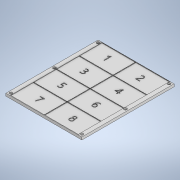
# Autodesk Inventor part: 8pos_slas_table
Saved by Autodesk Inventor 2020 (Build 240168000, 168)
## iProperties
Created: 2023-04-21
Part Number: 8pos_slas_table
Material: Generic
Document SubType Name: Modeling
Designer: Beaucage
Density: 1 g/cm^3
Appearance: Default
Author: Beaucage
Autodesk Inventor part; units mm, degrees
ref_plane "YZ Plane" through (0, 0, 0) normal (1, 0, 0) x (0, 1, 0)
ref_plane "XZ Plane" through (0, 0, 0) normal (0, 1, 0) x (-1, 0, 0)
ref_plane "XY Plane" through (0, 0, 0) normal (0, 0, 1) x (1, 0, 0)
sketch "Sketch1" plane through (0, 0, 0) normal (0, 1, 0) x (-1, 0, 0)
  line L0 (0, 0) -> (290, 0)
  line L1 (290, 0) -> (290, -351.8916)
  line L2 (290, -351.8916) -> (0, -351.8916)
  line L3 (0, -351.8916) -> (0, 0)
  dimension "d0" = 290
  dimension "d1" = 351.8916
  constraints: 8 end point, 2 parallel, 1 horizontal, 1 perpendicular
  measures "d0" distance of L1.end L2.end
  measures "d1" distance of L0.end L1.end
extrude "Extrusion1" add sketch "Sketch1" along normal blind 10
sketch "Sketch2" plane through (0, 10, 0) normal (0, 1, 0) x (1, 0, 0)
  line L0 (-290, 0) -> (0, 0) projected
  line L1 (0, 0) -> (-2, 0)
  line L2 (-2, 0) -> (-2, 2)
  line L3 (-2, 2) -> (0, 2)
  line L4 (0, 2) -> (0, 0)
  line L5 (0, 0) -> (0, 351.8916) projected
  line L6 (-2, 2) -> (0, 2)
  line L7 (0, 2) -> (0, 351.8916)
  line L8 (0, 351.8916) -> (-2, 351.8916)
  line L9 (-2, 351.8916) -> (-2, 2)
  line L10 (-290, 351.8916) -> (-290, 0) projected
  line L11 (0, 351.8916) -> (-290, 351.8916)
  line L12 (-290, 351.8916) -> (-290, 349.8916)
  line L13 (-290, 349.8916) -> (0, 349.8916)
  line L14 (0, 349.8916) -> (0, 351.8916)
  line L15 (0, 351.8916) -> (-290, 351.8916) projected
  line L16 (-290, 351.8916) -> (-288, 351.8916)
  line L17 (-288, 351.8916) -> (-288, 0)
  line L18 (-288, 0) -> (-290, 0)
  line L19 (-290, 0) -> (-290, 351.8916)
  line L20 (-290, 0) -> (0, 0)
  line L21 (0, 0) -> (0, 2)
  line L22 (0, 2) -> (-290, 2)
  line L23 (-290, 2) -> (-290, 0)
  line L24 (-2, 2) -> (-129.762, 2)
  line L25 (-2, 87.471) -> (-2, 2)
  line L26 (-131.762, 2) -> (-129.762, 2)
  line L27 (-288, 87.471) -> (-288, 89.471)
  line L28 (-2, 89.471) -> (-2, 87.471)
  line L29 (-262.0386, 2) -> (-134.2766, 2)
  line L30 (0, 2) -> (-15.7353, 2)
  line L31 (-15.7353, 2) -> (-144.5133, 2)
  line L32 (-144.5133, 2) -> (-144.5133, 88.487)
  line L33 (-144.5133, 88.487) -> (-15.7353, 88.487)
  line L34 (-15.7353, 88.487) -> (-15.7353, 2)
  line L35 (-144.5133, 88.487) -> (-146.5133, 88.487)
  line L36 (-146.5133, 88.487) -> (-146.5133, 2)
  line L37 (-146.5133, 2) -> (-144.5133, 2)
  line L38 (-144.5133, 2) -> (-144.5133, 88.487)
  point P0 (-288, 2)
  point P1 (-2, 349.8916)
  point P2 (-288, 349.8916)
  point P3 (-144.5133, 2)
  point P4 (-15.7353, 2)
  dimension "d4" = 2
  dimension "d5" = 2
  dimension "d6" = 2
  dimension "d7" = 2
  dimension "d8" = 2
  dimension "d13" = 2
  dimension "d14" = 2
  dimension "d17" = 127.762
  dimension "d19" = 15.7353
  dimension "d20" = 128.778
  dimension "d21" = 86.487
  dimension "d22" = 2
  constraints: 70 end point, 15 parallel, 8 horizontal, 7 perpendicular, 6 point on line
  measures "d4" distance of L2.end L3.end
  measures "d5" distance of L1.end L2.end
  measures "d6" distance of L12.end L11.end
  measures "d7" distance of L17.end L18.end
  measures "d8" distance of L6.end L20.end
  measures "d13" distance of L26.end L26.start
  measures "d14" distance of L27.start L27.end
  measures "d17" distance of L29.end L29.start
  measures "d19" distance of L6.end L30.end
  measures "d20" distance of L32.end L33.end
  measures "d21" distance of L31.end L32.end
  measures "d22" distance of L37.end L36.end
extrude "Extrusion4" cut sketch "Sketch2" against normal blind 2 contours L22 L32 L33 L34
pattern_linear "Rectangular Pattern1" count 2 spacing 129.762 along (-1, 0, 0) count 4 spacing 87.471 along (0, 0, -1) of "Extrusion4"
sketch "Sketch3" plane through (0, 10, 0) normal (0, 1, 0) x (1, 0, 0)
  line L0 (-290, 351.8916) -> (-290, 0) projected
  line L1 (-290, 0) -> (-280.475, 0)
  line L2 (-290, 0) -> (0, 0) projected
  line L3 (-280.475, 0) -> (-280.475, 9.525)
  line L4 (-290, 351.8916) -> (-280.475, 351.8916)
  line L5 (-280.475, 351.8916) -> (-280.475, 342.3666)
  line L6 (0, 0) -> (0, 351.8916) projected
  line L7 (0, 351.8916) -> (-9.525, 351.8916)
  line L8 (0, 351.8916) -> (-290, 351.8916) projected
  line L9 (-9.525, 351.8916) -> (-9.525, 342.3666)
  line L10 (0, 0) -> (-9.525, 0)
  line L11 (-9.525, 0) -> (-9.525, 9.525)
  line L12 (-290, 351.8916) -> (-290, 0) projected
  line L13 (-290, 175.9458) -> (-280.475, 175.9458)
  line L14 (0, 175.9458) -> (-9.525, 175.9458)
  dimension "d31" = 9.525
  dimension "d32" = 9.525
  dimension "d33" = 9.525
  dimension "d34" = 9.525
  dimension "d35" = 9.525
  dimension "d36" = 9.525
  constraints: 20 end point, 3 horizontal, 3 perpendicular, 3 point on line, 2 midpoint, 1 vertical
  measures "d31" distance of L0.end L1.end
  measures "d32" distance of L1.end L3.end
  measures "d33" distance of L0.start L4.end
  measures "d34" distance of L4.end L5.end
  measures "d35" distance of L6.end L7.end
  measures "d36" distance of L10.end L11.end
hole "Hole1" at (-280.475, 10, -342.3666) at (-9.525, 10, -342.3666) at (-9.525, 10, -9.525) at (-280.475, 10, -9.525) at (-280.475, 10, -175.9458) at (-9.525, 10, -175.9458) direction (0, -1, 0) diameter 6.7564 depth 9.9 counterbore diameter 11.1252 counterbore depth 6.35 clearance for "Socket Head Cap Screw" size "1/4" standard "Ansi Unified Screw Threads"
sketch "Sketch4" plane through (0, 8, 0) normal (0, 1, 0) x (1, 0, 0)
  line L0 (-94.0241, 322.1663) -> (-46.4018, 322.1663) construction
  line L1 (-46.4018, 322.1663) -> (-46.4018, 267.8366) construction
  line L2 (-46.4018, 267.8366) -> (-94.0241, 267.8366) construction
  line L3 (-94.0241, 267.8366) -> (-94.0241, 322.1663) construction
  line L4 (-224.5716, 324.4245) -> (-176.9493, 324.4245) construction
  line L5 (-176.9493, 324.4245) -> (-176.9493, 270.0949) construction
  line L6 (-176.9493, 270.0949) -> (-224.5716, 270.0949) construction
  line L7 (-224.5716, 270.0949) -> (-224.5716, 324.4245) construction
  line L8 (-224.5716, 324.4245) -> (-176.9493, 324.4245) construction
  line L9 (-176.9493, 324.4245) -> (-176.9493, 270.0949) construction
  line L10 (-176.9493, 270.0949) -> (-224.5716, 270.0949) construction
  line L11 (-224.5716, 270.0949) -> (-224.5716, 324.4245) construction
  line L12 (-223.2301, 237.2288) -> (-175.6078, 237.2288) construction
  line L13 (-175.6078, 237.2288) -> (-175.6078, 182.8992) construction
  line L14 (-175.6078, 182.8992) -> (-223.2301, 182.8992) construction
  line L15 (-223.2301, 182.8992) -> (-223.2301, 237.2288) construction
  line L16 (-92.8613, 183.1452) -> (-92.8613, 237.4748) construction
  line L17 (-92.8613, 237.4748) -> (-45.239, 237.4748) construction
  line L18 (-45.239, 237.4748) -> (-45.239, 183.1452) construction
  line L19 (-45.239, 183.1452) -> (-92.8613, 183.1452) construction
  line L20 (-91.7658, 148.6916) -> (-44.1436, 148.6916) construction
  line L21 (-44.1436, 148.6916) -> (-44.1436, 94.362) construction
  line L22 (-44.1436, 94.362) -> (-91.7658, 94.362) construction
  line L23 (-91.7658, 94.362) -> (-91.7658, 148.6916) construction
  line L24 (-220.3011, 93.2666) -> (-220.3011, 147.5962) construction
  line L25 (-220.3011, 147.5962) -> (-172.6789, 147.5962) construction
  line L26 (-172.6789, 147.5962) -> (-172.6789, 93.2666) construction
  line L27 (-172.6789, 93.2666) -> (-220.3011, 93.2666) construction
  line L28 (-216.9474, 3.3879) -> (-216.9474, 57.7176) construction
  line L29 (-216.9474, 57.7176) -> (-169.3252, 57.7176) construction
  line L30 (-169.3252, 57.7176) -> (-169.3252, 3.3879) construction
  line L31 (-169.3252, 3.3879) -> (-216.9474, 3.3879) construction
  line L32 (-89.2616, 4.3047) -> (-89.2616, 58.6343) construction
  line L33 (-89.2616, 58.6343) -> (-41.6393, 58.6343) construction
  line L34 (-41.6393, 58.6343) -> (-41.6393, 4.3047) construction
  line L35 (-41.6393, 4.3047) -> (-89.2616, 4.3047) construction
  spline S0 degree 2 poles (-87.6593, 39.9024) (-87.6593, 40.9156) (-87.0232, 42.9419) (-85.845, 44.7091) (-84.0779, 46.17) (-82.9705, 46.5941) knots 0 0 0 1 2 3 4 4 4
  spline S1 degree 2 poles (-82.9705, 46.5941) (-84.6198, 47.513) (-86.5755, 50.4111) (-86.5755, 52.1547) knots 0 0 0 1 2 2 2
  spline S2 degree 2 poles (-86.5755, 52.1547) (-86.5755, 53.5685) (-85.4916, 55.9247) (-83.5831, 57.6683) (-80.9441, 58.6343) (-79.4361, 58.6343) knots 0 0 0 1 2 3 4 4 4
  spline S3 degree 2 poles (-79.4361, 58.6343) (-77.881, 58.6343) (-75.2656, 57.6447) (-73.3571, 55.9247) (-72.2968, 53.5449) (-72.2968, 52.1547) knots 0 0 0 1 2 3 4 4 4
  spline S4 degree 2 poles (-72.2968, 52.1547) (-72.2968, 50.4111) (-74.2289, 47.513) (-75.8547, 46.5941) knots 0 0 0 1 2 2 2
  spline S5 degree 2 poles (-75.8547, 46.5941) (-74.7473, 46.17) (-73.0037, 44.7091) (-71.8256, 42.9419) (-71.1894, 40.9156) (-71.1894, 39.9024) knots 0 0 0 1 2 3 4 4 4
  spline S6 degree 2 poles (-71.1894, 39.9024) (-71.1894, 38.2295) (-72.3911, 35.4727) (-74.5823, 33.4935) (-77.5983, 32.4097) (-79.4361, 32.4097) knots 0 0 0 1 2 3 4 4 4
  spline S7 degree 2 poles (-79.4361, 32.4097) (-81.2269, 32.4097) (-84.2428, 33.4935) (-86.4341, 35.4727) (-87.6593, 38.2295) (-87.6593, 39.9024) knots 0 0 0 1 2 3 4 4 4
  spline S8 degree 2 poles (-84.502, 40.138) (-84.502, 38.9599) (-83.7951, 37.0514) (-82.4521, 35.7084) (-80.5671, 34.9779) (-79.4126, 34.9779) knots 0 0 0 1 2 3 4 4 4
  spline S9 degree 2 poles (-79.4126, 34.9779) (-78.3052, 34.9779) (-76.4202, 35.7084) (-75.0536, 37.0514) (-74.2996, 38.9835) (-74.2996, 40.138) knots 0 0 0 1 2 3 4 4 4
  spline S10 degree 2 poles (-74.2996, 40.138) (-74.2996, 41.1983) (-75.0065, 43.0598) (-76.3731, 44.497) (-78.2345, 45.2982) (-79.4126, 45.2982) knots 0 0 0 1 2 3 4 4 4
  spline S11 degree 2 poles (-79.4126, 45.2982) (-80.52, 45.2982) (-82.3578, 44.5442) (-83.7245, 43.1776) (-84.502, 41.269) (-84.502, 40.138) knots 0 0 0 1 2 3 4 4 4
  spline S12 degree 2 poles (-83.6066, 51.9191) (-83.6066, 51.0238) (-82.9469, 49.4922) (-81.7924, 48.3377) (-80.2844, 47.6779) (-79.4126, 47.6779) knots 0 0 0 1 2 3 4 4 4
  spline S13 degree 2 poles (-79.4126, 47.6779) (-78.5408, 47.6779) (-77.0092, 48.3377) (-75.8783, 49.4922) (-75.195, 51.0473) (-75.195, 51.9191) knots 0 0 0 1 2 3 4 4 4
  spline S14 degree 2 poles (-75.195, 51.9191) (-75.195, 52.838) (-75.8547, 54.4167) (-76.9857, 55.5477) (-78.5172, 56.2074) (-79.4126, 56.2074) knots 0 0 0 1 2 3 4 4 4
  spline S15 degree 2 poles (-79.4126, 56.2074) (-80.3551, 56.2074) (-81.8866, 55.5241) (-83.0176, 54.3696) (-83.6066, 52.8145) (-83.6066, 51.9191) knots 0 0 0 1 2 3 4 4 4
  spline S16 degree 2 poles (-199.0638, 56.0447) (-199.6293, 55.0315) (-201.2786, 52.0155) (-203.1165, 48.2691) (-205.0486, 43.9337) (-206.6979, 39.3391) (-207.9703, 34.6031) (-208.253, 32.3176) knots 0 0 0 1 2 3 4 5 6 6 6
  line L36 (-208.253, 32.3176) -> (-211.3632, 32.3176)
  spline S17 degree 2 poles (-211.3632, 32.3176) (-211.0569, 34.5795) (-209.7139, 39.3155) (-208.0409, 43.863) (-206.156, 48.0806) (-204.3888, 51.6385) (-202.9044, 54.3482) (-202.4803, 55.1022) knots 0 0 0 1 2 3 4 5 6 6 6
  line L37 (-202.4803, 55.1022) -> (-215.2038, 55.1022)
  line L38 (-215.2038, 55.1022) -> (-215.2038, 57.7176)
  line L39 (-215.2038, 57.7176) -> (-199.0638, 57.7176)
  line L40 (-199.0638, 57.7176) -> (-199.0638, 56.0447)
  spline S18 degree 2 poles (-203.1243, 129.9482) (-203.1243, 128.0867) (-204.3967, 125.0943) (-206.7529, 122.9266) (-210.0987, 121.7485) (-212.1251, 121.7485) knots 0 0 0 1 2 3 4 4 4
  spline S19 degree 2 poles (-212.1251, 121.7485) (-215.6829, 121.7485) (-217.403, 122.8088) knots 0 0 0 1 1 1
  line L41 (-217.403, 122.8088) -> (-217.403, 125.8955)
  spline S20 degree 2 poles (-217.403, 125.8955) (-214.8111, 124.2225) (-212.1015, 124.2225) knots 0 0 0 1 1 1
  spline S21 degree 2 poles (-212.1015, 124.2225) (-210.7113, 124.2225) (-208.4965, 125.0472) (-206.9414, 126.5081) (-206.1167, 128.558) (-206.1167, 129.7832) knots 0 0 0 1 2 3 4 4 4
  spline S22 degree 2 poles (-206.1167, 129.7832) (-206.1167, 132.2572) (-209.439, 135.0847) (-212.6199, 135.0847) knots 0 0 0 1 2 2 2
  spline S23 degree 2 poles (-212.6199, 135.0847) (-213.1147, 135.0847) (-214.2692, 135.0376) (-215.4002, 134.9905) (-216.4841, 134.9198) (-216.9082, 134.8726) knots 0 0 0 1 2 3 4 4 4
  line L42 (-216.9082, 134.8726) -> (-216.0599, 147.5962)
  line L43 (-216.0599, 147.5962) -> (-204.3024, 147.5962)
  line L44 (-204.3024, 147.5962) -> (-204.3024, 144.9808)
  line L45 (-204.3024, 144.9808) -> (-213.5388, 144.9808)
  line L46 (-213.5388, 144.9808) -> (-214.0572, 137.5116)
  spline S24 degree 2 poles (-214.0572, 137.5116) (-213.4681, 137.5587) (-212.1957, 137.6058) (-211.7009, 137.6058) knots 0 0 0 1 2 2 2
  spline S25 degree 2 poles (-211.7009, 137.6058) (-209.6982, 137.6058) (-206.4937, 136.5456) (-204.2789, 134.5899) (-203.1243, 131.7389) (-203.1243, 129.9482) knots 0 0 0 1 2 3 4 4 4
  spline S26 degree 2 poles (-73.6465, 130.9258) (-73.6465, 129.0644) (-74.8718, 125.9542) (-76.9924, 123.6922) (-79.9376, 122.4198) (-81.6577, 122.4198) knots 0 0 0 1 2 3 4 4 4
  spline S27 degree 2 poles (-81.6577, 122.4198) (-83.5662, 122.4198) (-86.5821, 124.0221) (-88.7027, 127.0145) (-89.8102, 131.3263) (-89.8102, 134.036) knots 0 0 0 1 2 3 4 4 4
  spline S28 degree 2 poles (-89.8102, 134.036) (-89.8102, 137.3583) (-88.3257, 142.754) (-85.6161, 146.6182) (-81.799, 148.6916) (-79.4428, 148.6916) knots 0 0 0 1 2 3 4 4 4
  spline S29 degree 2 poles (-79.4428, 148.6916) (-76.8039, 148.6916) (-75.2252, 147.9848) knots 0 0 0 1 1 1
  line L47 (-75.2252, 147.9848) -> (-75.2252, 145.228)
  spline S30 degree 2 poles (-75.2252, 145.228) (-77.1808, 146.2412) (-79.3721, 146.2412) knots 0 0 0 1 1 1
  spline S31 degree 2 poles (-79.3721, 146.2412) (-81.0686, 146.2412) (-83.8018, 144.7096) (-85.7339, 141.9293) (-86.7942, 137.9944) (-86.7942, 135.5911) knots 0 0 0 1 2 3 4 4 4
  line L48 (-86.7942, 135.5911) -> (-86.7235, 135.5911)
  spline S32 degree 2 poles (-86.7235, 135.5911) (-84.9564, 138.772) (-80.9272, 138.772) knots 0 0 0 1 1 1
  spline S33 degree 2 poles (-80.9272, 138.772) (-79.2543, 138.772) (-76.5918, 137.6174) (-74.6833, 135.544) (-73.6465, 132.6929) (-73.6465, 130.9258) knots 0 0 0 1 2 3 4 4 4
  spline S34 degree 2 poles (-76.6389, 130.5488) (-76.6389, 131.8918) (-77.2987, 134.0124) (-78.571, 135.4968) (-80.4089, 136.298) (-81.587, 136.298) knots 0 0 0 1 2 3 4 4 4
  spline S35 degree 2 poles (-81.587, 136.298) (-82.6473, 136.298) (-84.5087, 135.4733) (-85.8517, 134.0831) (-86.6057, 132.2217) (-86.6057, 131.185) knots 0 0 0 1 2 3 4 4 4
  spline S36 degree 2 poles (-86.6057, 131.185) (-86.6057, 129.8655) (-85.8753, 127.58) (-84.5087, 125.8835) (-82.6473, 124.8939) (-81.5163, 124.8939) knots 0 0 0 1 2 3 4 4 4
  spline S37 degree 2 poles (-81.5163, 124.8939) (-80.4324, 124.8939) (-78.6181, 125.7421) (-77.3458, 127.2265) (-76.6389, 129.3) (-76.6389, 130.5488) knots 0 0 0 1 2 3 4 4 4
  line L49 (-77.805, 237.4748) -> (-77.805, 220.6986)
  line L50 (-77.805, 220.6986) -> (-74.5299, 220.6986)
  line L51 (-74.5299, 220.6986) -> (-74.5299, 218.0361)
  line L52 (-74.5299, 218.0361) -> (-77.805, 218.0361)
  line L53 (-77.805, 218.0361) -> (-77.805, 212.0748)
  line L54 (-77.805, 212.0748) -> (-80.6796, 212.0748)
  line L55 (-80.6796, 212.0748) -> (-80.6796, 218.0361)
  line L56 (-80.6796, 218.0361) -> (-92.6021, 218.0361)
  line L57 (-92.6021, 218.0361) -> (-92.6021, 220.5572)
  spline S38 degree 2 poles (-92.6021, 220.5572) (-90.9527, 222.4422) (-87.5362, 226.7069) (-84.4496, 231.1131) (-81.8106, 235.4721) (-80.8917, 237.4748) knots 0 0 0 1 2 3 4 4 4
  line L58 (-80.8917, 237.4748) -> (-77.805, 237.4748)
  line L59 (-89.3269, 220.6986) -> (-80.6796, 220.6986)
  line L60 (-80.6796, 220.6986) -> (-80.6796, 233.1394)
  spline S39 degree 2 poles (-80.6796, 233.1394) (-81.9991, 230.8303) (-84.3789, 227.1782) (-86.523, 224.1858) (-88.4787, 221.7824) (-89.3269, 220.6986) knots 0 0 0 1 2 3 4 4 4
  spline S40 degree 2 poles (-206.336, 218.5911) (-206.336, 216.8711) (-207.632, 214.0672) (-209.9882, 212.0644) (-213.2869, 210.957) (-215.2661, 210.957) knots 0 0 0 1 2 3 4 4 4
  spline S41 degree 2 poles (-215.2661, 210.957) (-218.9182, 210.957) (-221.0624, 212.3472) knots 0 0 0 1 1 1
  line L61 (-221.0624, 212.3472) -> (-221.0624, 215.4574)
  spline S42 degree 2 poles (-221.0624, 215.4574) (-218.4705, 213.431) (-215.1718, 213.431) knots 0 0 0 1 1 1
  spline S43 degree 2 poles (-215.1718, 213.431) (-213.8288, 213.431) (-211.6846, 214.1143) (-210.1531, 215.3867) (-209.3284, 217.201) (-209.3284, 218.332) knots 0 0 0 1 2 3 4 4 4
  spline S44 degree 2 poles (-209.3284, 218.332) (-209.3284, 223.3036) (-216.3971, 223.3036) knots 0 0 0 1 1 1
  line L62 (-216.3971, 223.3036) -> (-218.5177, 223.3036)
  line L63 (-218.5177, 223.3036) -> (-218.5177, 225.7776)
  line L64 (-218.5177, 225.7776) -> (-216.5149, 225.7776)
  spline S45 degree 2 poles (-216.5149, 225.7776) (-210.2474, 225.7776) (-210.2474, 230.4429) knots 0 0 0 1 1 1
  spline S46 degree 2 poles (-210.2474, 230.4429) (-210.2474, 234.7783) (-215.0305, 234.7783) knots 0 0 0 1 1 1
  spline S47 degree 2 poles (-215.0305, 234.7783) (-217.7166, 234.7783) (-220.0728, 232.9641) knots 0 0 0 1 1 1
  line L65 (-220.0728, 232.9641) -> (-220.0728, 235.7915)
  spline S48 degree 2 poles (-220.0728, 235.7915) (-217.6459, 237.2288) (-214.3, 237.2288) knots 0 0 0 1 1 1
  spline S49 degree 2 poles (-214.3, 237.2288) (-212.6978, 237.2288) (-210.1295, 236.357) (-208.2681, 234.7548) (-207.255, 232.5164) (-207.255, 231.1733) knots 0 0 0 1 2 3 4 4 4
  spline S50 degree 2 poles (-207.255, 231.1733) (-207.255, 226.1546) (-212.3444, 224.7173) knots 0 0 0 1 1 1
  line L66 (-212.3444, 224.7173) -> (-212.3444, 224.6466)
  spline S51 degree 2 poles (-212.3444, 224.6466) (-211.0485, 224.5052) (-208.8336, 223.5392) (-207.255, 221.9841) (-206.336, 219.8635) (-206.336, 218.5911) knots 0 0 0 1 2 3 4 4 4
  line L67 (-211.7538, 298.459) -> (-214.6519, 298.459)
  line L68 (-214.6519, 298.459) -> (-214.6519, 320.4189)
  spline S52 degree 2 poles (-214.6519, 320.4189) (-214.9818, 320.0655) (-216.2777, 319.2173) (-217.9035, 318.3455) (-219.6706, 317.615) (-220.5424, 317.403) knots 0 0 0 1 2 3 4 4 4
  line L69 (-220.5424, 317.403) -> (-220.5424, 320.3482)
  spline S53 degree 2 poles (-220.5424, 320.3482) (-219.5764, 320.6074) (-217.4322, 321.5028) (-215.3588, 322.6338) (-213.5209, 323.859) (-212.8376, 324.4245) knots 0 0 0 1 2 3 4 4 4
  line L70 (-212.8376, 324.4245) -> (-211.7538, 324.4245)
  line L71 (-211.7538, 324.4245) -> (-211.7538, 298.459)
  spline S54 degree 2 poles (-80.3344, 315.0976) (-80.3344, 316.2522) (-81.0649, 317.9958) (-82.3372, 319.1503) (-84.0337, 319.7158) (-85.0233, 319.7158) knots 0 0 0 1 2 3 4 4 4
  spline S55 degree 2 poles (-85.0233, 319.7158) (-85.8716, 319.7158) (-87.4973, 319.2446) (-89.0524, 318.4434) (-90.4897, 317.3125) (-91.1023, 316.6056) knots 0 0 0 1 2 3 4 4 4
  line L72 (-91.1023, 316.6056) -> (-91.1023, 319.7394)
  spline S56 degree 2 poles (-91.1023, 319.7394) (-89.8771, 320.9175) (-86.8376, 322.1663) (-84.6699, 322.1663) knots 0 0 0 1 2 2 2
  spline S57 degree 2 poles (-84.6699, 322.1663) (-83.1148, 322.1663) (-80.4523, 321.2709) (-78.4966, 319.5273) (-77.3892, 316.9826) (-77.3892, 315.3332) knots 0 0 0 1 2 3 4 4 4
  spline S58 degree 2 poles (-77.3892, 315.3332) (-77.3892, 313.8253) (-78.0725, 311.3748) (-79.4862, 309.2306) (-81.6068, 307.2279) (-83.0441, 306.2147) knots 0 0 0 1 2 3 4 4 4
  spline S59 degree 2 poles (-83.0441, 306.2147) (-84.8348, 304.9423) (-87.1439, 303.128) (-88.5105, 301.5494) (-89.0524, 299.9707) (-89.0524, 298.9575) knots 0 0 0 1 2 3 4 4 4
  line L73 (-89.0524, 298.9575) -> (-76.4231, 298.9575)
  line L74 (-76.4231, 298.9575) -> (-76.4231, 296.3421)
  line L75 (-76.4231, 296.3421) -> (-92.092, 296.3421)
  line L76 (-92.092, 296.3421) -> (-92.092, 297.5909)
  spline S60 degree 2 poles (-92.092, 297.5909) (-92.092, 299.2403) (-91.3851, 301.7143) (-89.7593, 303.9527) (-87.1203, 306.1676) (-85.2118, 307.5813) knots 0 0 0 1 2 3 4 4 4
  spline S61 degree 2 poles (-85.2118, 307.5813) (-83.8216, 308.5709) (-81.9602, 310.3852) (-80.8293, 312.1759) (-80.3344, 314.0373) (-80.3344, 315.0976) knots 0 0 0 1 2 3 4 4 4
  point P0 (0, 0)
  constraints: 17 other
extrude "Extrusion5" cut sketch "Sketch4" against normal blind 2
body "Solid1"
